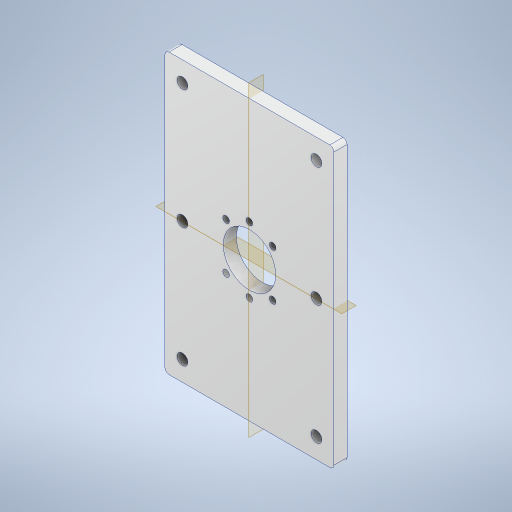
# Autodesk Inventor part: Z-Axis Nut Plate
Saved by Autodesk Inventor 2024 (Build 280153000, 153)
## iProperties
Created: 2024-12-31
Part Number: Z-Axis Nut Plate
Material: Aluminum 6061
Document SubType Name: Modeling
Designer: Ishaan
Density: 2.7 g/cm^3
Appearance: Aluminum - Flat
Author: Ishaan
Autodesk Inventor part; units mm, degrees
ref_plane "XY Plane" through (0, 0, 0) normal (0, 0, 1) x (1, 0, 0)
sketch "Sketch1" plane through (0, 0, 0) normal (0, 0, 1) x (1, 0, 0)
  line L0 (41, -67.75) -> (-41, -67.75)
  line L1 (-41, -67.75) -> (-41, 67.75)
  line L2 (-41, 67.75) -> (41, 67.75)
  line L3 (41, 67.75) -> (41, -67.75)
  line L4 (41, -67.75) -> (-41, 67.75) construction
  line L5 (-41, -67.75) -> (41, 67.75) construction
  circle A0 centre (0, 0) radius 12.75
  line L6 (11.3137, -11.3137) -> (-11.3137, -11.3137) construction
  line L7 (-11.3137, -11.3137) -> (-11.3137, 11.3137) construction
  line L8 (-11.3137, 11.3137) -> (11.3137, 11.3137) construction
  line L9 (11.3137, 11.3137) -> (11.3137, -11.3137) construction
  line L10 (11.3137, -11.3137) -> (-11.3137, 11.3137) construction
  line L11 (-11.3137, -11.3137) -> (11.3137, 11.3137) construction
  circle A1 centre (0, 0) radius 16 construction
  line L12 (0, 16) -> (0, -16) construction
  dimension "d0" = 82
  dimension "d1" = 135.5
  dimension "d2" = 25.5
  dimension "d3" = 32
  dimension "d4" = 0
  constraints: 26 end point, 8 coincident, 6 midpoint, 4 parallel, 3 perpendicular, 3 point on circle, 2 centre point, 2 horizontal, 1 vertical
  measures "d0" distance of L1.end L2.end
  measures "d1" distance of L0.end L1.end
  measures "d2" diameter of A0
  measures "d3" diameter of A1
  measures "d4" distance of point (0, 0) point (0, 0)
extrude "Extrusion1" add sketch "Sketch1" along normal blind 6.35
hole "Hole1" at (0, 16, 0) at (11.3137, 11.3137, 0) at (-11.3137, 11.3137, 0) at (11.3137, -11.3137, 0) at (0, -16, 0) at (-11.3137, -11.3137, 0) direction (0, 0, 1) diameter 3.242 end through all thread size "M4x0.7" class "6H" standard "ANSI Metric M Profile"
fillet "Fillet1" radius 2 4 edges at (41, 67.75, 3.175) (-41, 67.75, 3.175) (-41, -67.75, 3.175) (41, -67.75, 3.175)
sketch "Sketch2" plane through (0, 0, 6.35) normal (0, 0, 1) x (1, 0, 0)
  line L0 (32.5, -58) -> (-32.5, -58) construction
  line L1 (-32.5, -58) -> (-32.5, 58) construction
  line L2 (-32.5, 58) -> (32.5, 58) construction
  line L3 (32.5, 58) -> (32.5, -58) construction
  line L4 (32.5, -58) -> (-32.5, 58) construction
  line L5 (-32.5, -58) -> (32.5, 58) construction
  point P0 (0, 0)
  point P1 (32.5, 0)
  point P2 (-32.5, 0)
  dimension "d15" = 65
  dimension "d16" = 116
  constraints: 12 end point, 4 coincident, 4 midpoint, 2 parallel, 1 horizontal, 1 perpendicular
  measures "d15" distance of L1.end L2.end
  measures "d16" distance of L0.end L1.end
hole "Hole2" at (-32.5, 58, 6.35) at (32.5, 58, 6.35) at (32.5, 0, 6.35) at (32.5, -58, 6.35) at (-32.5, -58, 6.35) at (-32.5, 0, 6.35) direction (0, 0, -1) diameter 5.3 end through all
body "Solid1"
